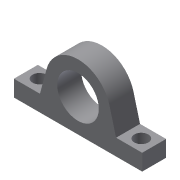
# Autodesk Inventor part: omni wheel shaft holder low channel side attach
Saved by Autodesk Inventor 2018 (Build 220112000, 112)
## iProperties
Created: 2019-02-06
Part Number: omni wheel shaft holder low channel side attach
Material: Generic
Document SubType Name: Modeling
Designer: ball
Density: 1 g/cm^3
Appearance: Default
Author: ball
Autodesk Inventor part; units mm, degrees
ref_plane "YZ Plane" through (0, 0, 0) normal (1, 0, 0) x (0, 1, 0)
ref_plane "XZ Plane" through (0, 0, 0) normal (0, 1, 0) x (-1, 0, 0)
ref_plane "XY Plane" through (0, 0, 0) normal (0, 0, 1) x (1, 0, 0)
sketch "Sketch1" plane through (0, 0, 0) normal (0, 0, 1) x (1, 0, 0)
  circle A0 centre (0, 0) radius 6.477
  arc A1 (9.8184, 2.6122) -> (-9.8184, 2.6122) centre (0, 0) ccw
  line L0 (0, -10.16) -> (-20, -10.16)
  line L1 (-20, -10.16) -> (-20, -5.08)
  line L2 (0, -5.08) -> (0, -10.16)
  line L3 (0, -10.16) -> (20, -10.16)
  line L4 (20, -10.16) -> (20, -5.08)
  line L5 (0, -5.08) -> (0, -10.16)
  line L6 (-16, -5.08) -> (-16, -10.16) construction
  line L7 (-19.5, -5.08) -> (-19.5, -10.16) construction
  line L8 (-12.5, -5.08) -> (-12.5, -10.16) construction
  line L9 (-11.865, -5.08) -> (-11.865, -10.16) construction
  line L10 (-11.865, -5.08) -> (-9.8184, 2.6122)
  line L11 (16, -5.08) -> (16, -10.16) construction
  line L12 (12.5, -5.08) -> (12.5, -10.16) construction
  line L13 (11.865, -5.08) -> (11.865, -10.16) construction
  line L14 (11.865, -5.08) -> (9.8184, 2.6122)
  line L15 (20, -5.08) -> (11.865, -5.08)
  line L16 (-20, -5.08) -> (-11.865, -5.08)
  dimension "d0" = 12.954
  dimension "d1" = 20.32
  dimension "d3" = 5.08
  dimension "d5" = 5.08
  dimension "d6" = 16
  dimension "d7" = 3.5
  dimension "d8" = 3.5
  dimension "d9" = 0.635
  dimension "d10" = 16
  dimension "d11" = 3.5
  dimension "d12" = 0.635
  constraints: 34 end point, 12 point on line, 9 perpendicular, 4 parallel, 2 centre point, 2 coincident, 2 horizontal, 2 point on circle, 2 tangent
  measures "d0" diameter of A0
  measures "d1" diameter of A1
  measures "d3" distance of L0.end L1.end
  measures "d5" distance of L4.end L3.end
  measures "d6" distance from line of point (0, 0) L6
  measures "d7" distance between parallel lines of L6 L7
  measures "d8" distance between parallel lines of L8 L6
  measures "d9" distance between parallel lines of L9 L8
  measures "d10" distance from line of L11 point (0, 0)
  measures "d11" distance between parallel lines of L11 L12
  measures "d12" distance between parallel lines of L12 L13
ref_plane "Work Plane1" through (-6.9215, -6.9215, 7.4676) normal (0, 0, -1) x (0, 1, 0)
extrude "Extrusion1" add sketch "Sketch1" along normal up to surface (7.4676 mm away)
sketch "Sketch2" plane through (11.865, -5.08, 0) normal (0, 1, 0) x (1, 0, 0)
  line L0 (8.135, 0) -> (8.135, -7.4676) construction
  line L1 (8.135, -3.4676) -> (0, -3.4676) construction
  line L2 (8.135, -7.4676) -> (0, -7.4676) construction
  line L3 (8.135, 0) -> (0, 0) construction
  line L4 (4.135, 0) -> (4.135, -7.4676) construction
  line L5 (-31.75, -3.4676) -> (-23.73, -3.4676) construction
  line L6 (-23.73, 0) -> (-23.73, -7.4676) construction
  line L7 (-23.73, -7.4676) -> (-31.865, -7.4676) construction
  line L8 (-31.865, -7.4676) -> (8.135, -7.4676) construction
  line L9 (-27.865, -7.4676) -> (-27.865, 0) construction
  line L10 (-31.865, 0) -> (-31.865, -7.4676) construction
  circle A0 centre (-27.865, -3.4676) radius 2.1844
  circle A1 centre (4.135, -3.7338) radius 2.1844
  point P0 (-11.865, 0)
  dimension "d15" = 4
  dimension "d16" = 4
  dimension "d17" = 4
  dimension "d18" = 4
  dimension "d19" = 4.3688
  dimension "d20" = 4.3688
  constraints: 8 end point, 6 point on line, 2 centre point, 2 perpendicular, 1 horizontal, 1 midpoint
  measures "d15" distance between parallel lines of L1 L2
  measures "d16" distance between parallel lines of L4 L0
  measures "d17" distance between parallel lines of L7 L5
  measures "d18" distance between parallel lines of L10 L9
  measures "d19" diameter of A0
  measures "d20" diameter of A1
hole "Hole1" at (-16, -5.08, 3.4676) at (16, -5.08, 3.7338) direction (0, -1, 0) diameter 4.3688 end through all
body "Solid1"
